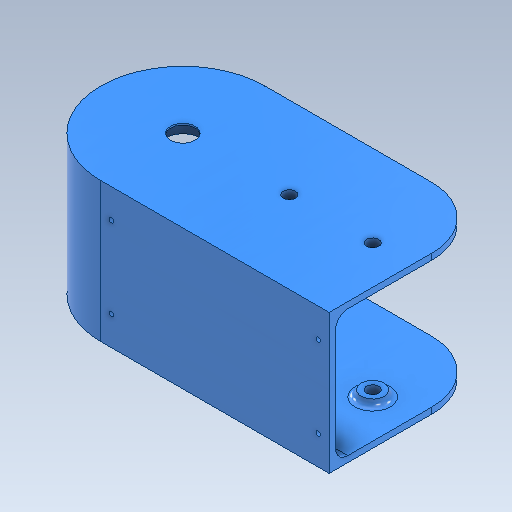
# Autodesk Inventor part: obudowa przekładni
Saved by Autodesk Inventor 2021 (Build 250183000, 183)
## iProperties
Created: 2021-06-25
Part Number: obudowa przekładni
Material: Generic
Document SubType Name: Modeling
Designer: Łukasz
Density: 1 g/cm^3
Appearance: Cyan
Author: Łukasz
Autodesk Inventor part; units mm, degrees
ref_plane "YZ Plane" through (0, 0, 0) normal (1, 0, 0) x (0, 1, 0)
ref_plane "XZ Plane" through (0, 0, 0) normal (0, 1, 0) x (-1, 0, 0)
sketch "Sketch1" plane through (0, 0, 0) normal (0, 1, 0) x (-1, 0, 0)
  circle A0 centre (0, 0) radius 11
  line L0 (0, -45) -> (-3.931, -45)
  line L1 (-3.2842, 50) -> (0, 50)
  line L2 (37.8352, 0) -> (26.6415, 27.0241)
  line L3 (26.6415, 27.0241) -> (-0.6792, 48)
  line L4 (-0.6792, 48) -> (-130, 48)
  line L5 (-130, -43) -> (-0.5468, -43)
  line L6 (-0.5468, -43) -> (26.692, -26.9021)
  line L7 (26.692, -26.9021) -> (37.8352, 0)
  line L8 (-130, 48) -> (-130, -43)
  line L9 (28.2843, -28.2843) -> (25.4178, -29.9783)
  line L10 (3.3842, -43) -> (0, -45)
  line L11 (40, 0) -> (38.9176, -2.6131)
  line L12 (29.5585, -25.2081) -> (28.2843, -28.2843)
  line L13 (28.2843, 28.2843) -> (29.8157, 24.587)
  line L14 (38.9176, 2.6131) -> (40, 0)
  line L15 (0, 50) -> (2.605, 48)
  line L16 (25.11, 30.7214) -> (28.2843, 28.2843)
  circle A1 centre (-69.5, 0) radius 4
  line L17 (1.9138, -52) -> (-130, -52)
  line L18 (-130, 57) -> (2.3773, 57)
  line L19 (2.3773, 57) -> (34.034, 32.695)
  line L20 (34.034, 32.695) -> (47.5767, 0)
  line L21 (47.5767, 0) -> (33.8573, -33.1217)
  line L22 (33.8573, -33.1217) -> (1.9138, -52)
  line L23 (-130, -52) -> (-130, -43)
  line L24 (-130, 48) -> (-130, 57)
  line L25 (-139, -45) -> (-139, -43)
  line L26 (-139, 48) -> (-139, 50)
  circle A2 centre (-123.9, 0) radius 4
  line L27 (-130, -52) -> (-139, -52)
  line L28 (-139, -52) -> (-139, 57)
  line L29 (-139, 57) -> (-130, 57)
  line L30 (-130, 57) -> (-130, -52)
  line L31 (-130, 52.0352) -> (-139, 52.0352)
  arc A3 (0, -53.0352) -> (8.4168, 52.3631) centre (0, 0) ccw
  line L32 (8.4168, 52.3631) -> (-139, 52.3631)
  line L33 (0, -53.0352) -> (-139, -53.0352)
  line L34 (-139, -53.0352) -> (-139, -52)
  arc A4 (-20.0914, 48) -> (-29.3029, -43) centre (0, 0) ccw
  arc A5 (-1.9138, -52) -> (1.9138, -52) centre (0, 0) ccw
  line L35 (-139, 52.3631) -> (-159, 52.3631)
  line L36 (-159, 52.3631) -> (-159, -52.0352)
  line L37 (-159, -52.0352) -> (-139, -52.0352)
  line L38 (-139, -52.0352) -> (-139, 52.3631)
  line L39 (-159, -52.0352) -> (-139, -52.0352)
  line L40 (-139, -52.0352) -> (-139, -53.0352)
  line L41 (-139, -53.0352) -> (-159, -53.0352)
  line L42 (-159, -53.0352) -> (-159, -52.0352)
  line L43 (-159, -53.0352) -> (-149, -53.0352)
  line L44 (-149, -53.0352) -> (-149, 52.3631)
  line L45 (-149, 52.3631) -> (-159, 52.3631)
  line L46 (-159, 52.3631) -> (-159, -53.0352)
  point P0 (0, 52.0352)
  dimension "d7" = 8
  dimension "d8" = 69.5
  dimension "d13" = 22
  dimension "d14" = 9
  dimension "d20" = 8
  dimension "d21" = 54.4
  dimension "d29" = 20
  dimension "d53" = 10
  constraints: 94 end point, 23 point on line, 9 parallel, 9 perpendicular, 6 centre point, 6 point on circle, 4 horizontal, 1 coincident, 1 midpoint, 1 tangent, 3 other
  measures "d7" diameter of A1
  measures "d8" distance of point (0, 0) A1.centre
  measures "d13" diameter of A0
  measures "d14" distance between parallel lines of L5 L17
  measures "d20" diameter of A2
  measures "d21" distance of A1.centre A2.centre
  measures "d29" distance of L37.end L36.end
  measures "d53" distance of L45.end L44.end
extrude "Extrusion1" add sketch "Sketch1" along normal blind 4 contours L7 L6 L5 A4 L4 L3 L2 | L2 L3 L4 L24 L32 L19 L20 L21 L22 L17 L23 L5 L6 L7 | A4 L5 L8 L4 | L8 L23 L27 L28 L25 L26 L31 L24 | L31 L28 L32 L24 | L17 A5 L22 L21 L20 L19 A3 L33 L34 L27 | L28 L26 L25 L34 L37 L44 L35 | L34 L41 L44 L37
sketch "Sketch2" plane through (0, 4, 0) normal (0, 1, 0) x (1, 0, 0)
  circle A0 centre (0, 0) radius 11 projected
  circle A1 centre (0, 0) radius 18
  circle A2 centre (69.5, 0) radius 4 projected
  circle A3 centre (69.5, 0) radius 7.5
  circle A4 centre (123.9, 0) radius 4 projected
  circle A5 centre (123.9, 0) radius 7.5
  dimension "d3" = 36
  dimension "d9" = 15
  dimension "d22" = 15
  constraints: 3 centre point, 3 coincident
  measures "d3" diameter of A1
  measures "d9" diameter of A3
  measures "d22" diameter of A5
extrude "Extrusion2" add sketch "Sketch2" along normal blind 4
sketch "Sketch3" plane through (0, 4, 0) normal (0, 1, 0) x (1, 0, 0)
  point P0 (0, 0)
fillet "Fillet3" radius 4 3 edges at (62, 4, 0) (-18, 4, 0) (116.4, 4, 0)
ref_plane "Work Plane1" through (0, 45.5, 0) normal (0, -1, 0) x (1, 0, 0)
mirror "Mirror1" about plane through (0, 45.5, 0) normal (0, -1, 0) of "Extrusion1", "Extrusion2", "Fillet3"
sketch "Sketch4" plane through (0, 0, 0) normal (0, -1, 0) x (1, 0, 0)
  point P0 (0, 0)
sketch "Sketch5" plane through (0, 0, 0) normal (0, -1, 0) x (1, 0, 0)
  circle A0 centre (0, 0) radius 8
  circle A1 centre (0, 0) radius 11 projected
  dimension "d15" = 16
  constraints: 1 centre point, 1 coincident
  measures "d15" diameter of A0
extrude "Extrusion3" add sketch "Sketch5" against normal blind 1
sketch "Sketch6" plane through (-2.3773, 91, 57) normal (0, 1, 0) x (1, 0, 0)
  circle A0 centre (2.3773, 57) radius 11 projected
  circle A1 centre (2.3773, 57) radius 8 projected
extrude "Extrusion4" add sketch "Sketch6" against normal blind 1
sketch "Sketch12" plane through (-8.4168, 91, 52.3631) normal (0, 1, 0) x (1, 0, 0)
  circle A0 centre (8.4168, 52.3631) radius 8 projected
  circle A1 centre (8.4168, 52.3631) radius 53.5
  line L0 (157.4168, 119.5335) -> (157.4168, -33.9038)
  line L1 (157.4168, 0) -> (157.4168, 105.3983) projected
  line L2 (8.4168, -1.1369) -> (157.4168, -1.1369)
  line L3 (8.4168, -1.1369) -> (157.4168, -1.1369) construction
  line L4 (8.4168, 105.8631) -> (157.4168, 105.8631)
  line L5 (-24.14, 81.9212) -> (153.427, 81.9212)
  line L6 (153.427, 81.9212) -> (153.427, 15.5578)
  line L7 (153.427, 15.5578) -> (-24.14, 15.5578)
  line L8 (-24.14, 15.5578) -> (-24.14, 81.9212)
  dimension "d54" = 107
  dimension "d55" = 0
  constraints: 16 end point, 3 coincident, 2 collinear, 2 horizontal, 2 parallel, 2 perpendicular, 2 point on circle, 2 point on line, 1 centre point
  measures "d54" diameter of A1
  measures "d55" distance between parallel lines of L2 L3
extrude "Extrusion8" add sketch "Sketch12" against normal up to surface (4 mm away) contours A1 L5 L8 L7 | L4 L0 L2 A1 L7 L6 L5 picked at (-30.4403, 45.067)
mirror "Mirror2" about plane through (0, 45.5, 0) normal (0, -1, 0) of "Extrusion8"
sketch "Sketch7" plane through (0, 4, 0) normal (0, 1, 0) x (1, 0, 0)
  line L0 (130, -52.0352) -> (139, -52.0352) projected
  arc A0 (0, 50.0352) -> (-8.1737, -49.3631) centre (0, 0) ccw
  line L1 (-8.1737, -49.3631) -> (139, -49.3631)
  line L2 (139, 52.0352) -> (139, 53.0352) projected
  line L3 (139, -49.3631) -> (139, -52.3631)
  line L4 (-53.0352, 0) -> (-50.0352, 0)
  line L5 (0, 50.0352) -> (139, 50.0352)
  line L6 (139, 53.0352) -> (0, 53.0352) projected
  line L7 (-8.4168, -52.3631) -> (149, -52.3631) projected
  line L8 (139, -49.3631) -> (159, -49.3631)
  line L9 (159, -49.3631) -> (159, -52.3631)
  line L10 (159, -52.3631) -> (139, -52.3631)
  line L11 (139, -52.3631) -> (139, -49.3631)
  line L12 (149, -52.3631) -> (149, 53.0352) projected
  line L13 (0, -53.5) -> (149, -53.5) projected
  arc A1 (0, 53.5) -> (0, -53.5) centre (0, 0) ccw projected
  line L14 (149, -53.5) -> (149, -52.3631)
  line L15 (-50.0352, 0) -> (-53.5, 0)
  point P0 (149, -49.3631)
  point P1 (149, 53.5)
  constraints: 20 end point, 4 point on circle, 2 horizontal, 2 parallel, 2 perpendicular, 1 centre point, 1 collinear, 1 point on line, 1 vertical
extrude "Extrusion5" add sketch "Sketch7" along normal up to surface (83 mm away) contours A0 L1 L3 L7 L14 L13 A1 L15 L4 | L8 L12 L7 L3
fillet "Fillet6" radius 40 2 edges at (149, 89, -53.5) (149, 2, -53.5)
sketch "Sketch10" plane through (159, 4, 49.3631) normal (0, 0, -1) x (-1, 0, 0)
  circle A0 centre (152.1737, 68) radius 1.5
  line L0 (167.1737, 0) -> (167.1737, 83) projected
  line L1 (10, 83) -> (159, 83) projected
  circle A1 centre (152.1737, 15) radius 1.5
  circle A2 centre (17.1737, 68) radius 1.5
  circle A3 centre (17.1737, 15) radius 1.5
  point P0 (159, -4)
  point P1 (45, 83)
  dimension "d34" = 3
  dimension "d35" = 15
  dimension "d36" = 15
  dimension "d39" = 53
  dimension "d42" = 135
  constraints: 4 centre point, 1 horizontal, 1 vertical, 6 other
  measures "d34" diameter of A0
  measures "d35" distance from line of L0 A0.centre
  measures "d36" distance from line of L1 A0.centre
  measures "d39" distance of A0.centre A1.centre
  measures "d42" distance of A0.centre A2.centre
extrude "Extrusion6" cut sketch "Sketch10" against normal up to surface (4.1369 mm away)
sketch "Sketch11" plane through (159, 4, 49.3631) normal (0, 0, -1) x (-1, 0, 0)
  circle A0 centre (152.1737, 68) radius 1.5 projected
  circle A1 centre (152.1737, 68) radius 4
  circle A2 centre (152.1737, 15) radius 1.5 projected
  circle A3 centre (152.1737, 15) radius 4
  circle A4 centre (17.1737, 68) radius 1.5 projected
  circle A5 centre (17.1737, 68) radius 4
  circle A6 centre (17.1737, 15) radius 1.5 projected
  circle A7 centre (17.1737, 15) radius 4
  point P0 (159, -4)
  dimension "d47" = 8
  dimension "d48" = 8
  dimension "d49" = 8
  dimension "d50" = 8
  constraints: 4 centre point, 4 coincident
  measures "d47" diameter of A1
  measures "d48" diameter of A3
  measures "d49" diameter of A5
  measures "d50" diameter of A7
extrude "Extrusion7" cut sketch "Sketch11" against normal blind 1
fillet "Fillet7" radius 8 2 edges at (70.4132, 4, 49.3631) (70.4132, 87, 49.3631)
body "Solid1"
